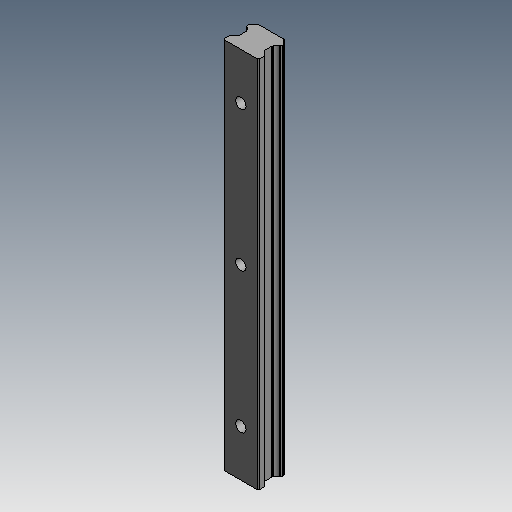
# Autodesk Inventor part: C-SXR24-160_r
Saved by Autodesk Inventor 2020 (Build 240168000, 168)
## iProperties
Part Number: C-SXR24-160_r
Material: 一般
Catalog Web Link: www.cadenas.de
Description: C-SXR, C-SX2R, C-SXRL, C-SX2RL_rail-C-VALUE Linear Guides for Heavy Load
Vendor: MISUMI
Document SubType Name: Modeling
Designer: partserver
Manufacturer: MISUMI
Mass: 25.7237 g
Surface Area: 100.566 cm^2
Volume: 25.7237 cm^3
Density: 1 g/cm^3
Appearance: PSOLRGB-192-192-192
Category: PARTsolutions
Company: MISUMI
PSOL_IDENT_0: {$CADENAS_DATA\23d-libs\misumi\metric\06_linear_guides\06_cn\c_sxr\c_sxr_rail.prj},208 {VTYP=3D},{NB=
PSOL_IDENT_1: C-SXR24-160_r},{LINA=C-SXR24-160},{NN=C-SXR, C-SX2R, C-SXRL, C-SX2RL_rail},{DATE=20.05.2021 06:43:21
PSOL_IDENT_2: },{GEOMDATE=11.06.2020 08:16:10},{VERSION=},{LINEID=10},{WBVAR=NOB,LT,LS,ALT},{WBNUMERIC=LS}  {NB=C-
PSOL_IDENT_3: SXR24-160_r},{LINA=C-SXR24-160},{KT=DUMMY},{PN=C-SXR24-160},{TYPE=C-SX},{H=24},{NOB=},{LT=},{LS=160}
PSOL_IDENT_4: ,{LALG=[100,160,220,280,340,400,460,520,580,640,700,760,820,880,940,1000,1060,1120,1180,1240,1300,13
PSOL_IDENT_5: 60,1420,1480]},{LSALG=[100,160,220,280,340,400,460,520,580,640,700,760,820,880,940,1000,1060,1120,11
PSOL_IDENT_6: 80,1240,1300,1360,1420,1480]},{LALG0=[110:150/10],[170:210/10],[230:270/10],[290:330/10],[350:390/10
PSOL_IDENT_7: ],[410:450/10],[470:510/10],[530:570/10],[590:630/10],[650:690/10],[710:750/10],[770:810/10],[830:87
PSOL_IDENT_8: 0/10],[890:930/10],[950:990/10],[1010:1050/10],[1070:1110/10],[1130:1170/10],[1190:1230/10],[1250:12
PSOL_IDENT_9: 90/10],[1310:1350/10],[1370:1410/10],[1430:1470/10]},{LMIN=110},{LMAX=1470},{L1=55.9},{E=7.0},{H1=13
PSOL_IDENT_10: .0},{W1=15},{W2=9.5},{CAA=0.5},{DD1=4.5},{DD2=7.5},{HH=6.0},{DDH=4.5x7.5x6},{F=60},{G=20},{LW1=7.217
PSOL_IDENT_11: },{LW2=11.000},{LH1=8.221},{LH2=4.659},{LH3=3.221},{LH4=4.700},{LC1=0.300},{LC2=2.000},{LC3=0.500},{
PSOL_IDENT_12: LR1=1.431},{LR2=0.300},{LR3=0.300},{LR4=0.300},{M=3},{ALT=},{ALTALG= '','Not applicable' },{NL=0},{C
PSOL_IDENT_13: IFCP=0}
NB: C-SXR24-160_r
NN: C-SXR, C-SX2R, C-SXRL, C-SX2RL_rail
NT: C-VALUE Linear Guides for Heavy Load
NBSYN: $PN._r
LINA: C-SXR24-160
CATALOG: Misumi
PN: C-SXR24-160
H: 24
NOB: 1
LT: Selectable
LS: 160
H1: 13
W1: 15
W2: 9.5
CAA: 0.5
DDH: 4.5x7.5x6
F: 60
G: 20
ALT: Not applicable
SUPPLIER: MISUMI
ARTICLENO: C-SXR24-160_r
BOMINFO: C-SXR24-160
CREATOR: CADENAS GmbH
Title: C-SXR24-160
Author: Cadenas PARTsolutions
Comments: C-VALUE Linear Guides for Heavy Load
Autodesk Inventor part; units mm, degrees
sketch "Sketch_2" plane through (0, 0, 0) normal (0, 0, 1) x (1, 0, 0)
  line L0 (-7.5, 10.787) -> (-7.5, 10.313)
  line L1 (-7.5, 10.313) -> (-7.2658, 9.8108)
  arc A0 (-7.2658, 9.8108) -> (-7.0326, 9.6401) centre (-6.9939, 9.9376) ccw
  arc A1 (-5.7891, 8.3153) -> (-7.0326, 9.6401) centre (-7.217, 8.221) ccw
  arc A2 (-5.7891, 8.3153) -> (-5.7019, 8.1229) centre (-5.4898, 8.335) ccw
  line L2 (-5.7019, 8.1229) -> (-5.5879, 8.0089)
  arc A3 (-5.5, 7.7967) -> (-5.5879, 8.0089) centre (-5.8, 7.7967) ccw
  line L3 (-5.5, 7.7967) -> (-5.5, 4.8243)
  arc A4 (-5.5879, 4.6121) -> (-5.5, 4.8243) centre (-5.8, 4.8243) ccw
  line L4 (-5.5879, 4.6121) -> (-7.4121, 2.7879)
  arc A5 (-7.4121, 2.7879) -> (-7.5, 2.5757) centre (-7.2, 2.5757) ccw
  line L5 (-7.5, 2.5757) -> (-7.5, 0.5)
  line L6 (-7.5, 0.5) -> (-7, 0)
  line L7 (-7, 0) -> (7, 0)
  line L8 (7, 0) -> (7.5, 0.5)
  line L9 (7.5, 0.5) -> (7.5, 2.5757)
  arc A6 (7.5, 2.5757) -> (7.4121, 2.7879) centre (7.2, 2.5757) ccw
  line L10 (7.4121, 2.7879) -> (5.5879, 4.6121)
  arc A7 (5.5, 4.8243) -> (5.5879, 4.6121) centre (5.8, 4.8243) ccw
  line L11 (5.5, 4.8243) -> (5.5, 7.7967)
  arc A8 (5.5879, 8.0089) -> (5.5, 7.7967) centre (5.8, 7.7967) ccw
  line L12 (5.5879, 8.0089) -> (5.7019, 8.1229)
  arc A9 (5.7019, 8.1229) -> (5.7891, 8.3153) centre (5.4898, 8.335) ccw
  arc A10 (7.0326, 9.6401) -> (5.7891, 8.3153) centre (7.217, 8.221) ccw
  arc A11 (7.0326, 9.6401) -> (7.2658, 9.8108) centre (6.9939, 9.9376) ccw
  line L13 (7.2658, 9.8108) -> (7.5, 10.313)
  line L14 (7.5, 10.313) -> (7.5, 10.787)
  line L15 (7.5, 10.787) -> (7.2653, 11.2903)
  arc A12 (7.2653, 11.2903) -> (7.0322, 11.461) centre (6.9934, 11.1635) ccw
  arc A13 (5.7938, 12.7312) -> (7.0322, 11.461) centre (7.217, 12.88) ccw
  arc A14 (5.7938, 12.7312) -> (5.4954, 13) centre (5.4954, 12.7) ccw
  line L16 (5.4954, 13) -> (-5.4954, 13)
  arc A15 (-5.4954, 13) -> (-5.7938, 12.7312) centre (-5.4954, 12.7) ccw
  arc A16 (-7.0322, 11.461) -> (-5.7938, 12.7312) centre (-7.217, 12.88) ccw
  arc A17 (-7.0322, 11.461) -> (-7.2653, 11.2903) centre (-6.9934, 11.1635) ccw
  line L17 (-7.2653, 11.2903) -> (-7.5, 10.787)
  constraints: 36 end point, 36 point on circle, 18 centre point
extrude "Extrusion1" add sketch "Sketch_2" along normal mid plane 160
sketch "Sketch2" plane through (-5.4954, 13, 80) normal (0, 1, 0) x (1, 0, 0)
  point P0 (5.4954, 20)
hole "Hole1" at (0, 13, 60) direction (0, -1, 0) diameter 4.5 depth 13 counterbore diameter 7.5 counterbore depth 6
pattern_linear "Rectangular Pattern1" count 3 spacing 60 along (0, 0, -1) of "Hole1"
ref_plane "to_block_1_XY" through (0, 13, 0) normal (0, 0, -1) x (1, 0, 0)
ref_plane "to_block_1_YZ" through (0, 13, 0) normal (1, 0, 0) x (0, -1, 0)
ref_plane "to_block_1_ZX" through (0, 13, 0) normal (0, -1, 0) x (0, 0, -1)
body "Solid1"
